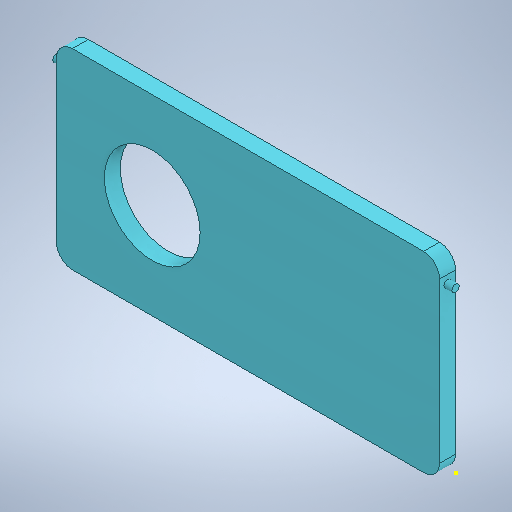
# Autodesk Inventor part: Puerta
Saved by Autodesk Inventor 2025.2 (Build 292293000, 293)
## iProperties
Created: 2024-11-26
Part Number: Puerta
Material: Plástico ABS
Document SubType Name: Modeling
Designer: usuario
Density: 1.06 g/cm^3
Appearance: Azul cadete
Author: usuario
Autodesk Inventor part; units mm, degrees
ref_plane "YZ Plane" through (0, 0, 0) normal (1, 0, 0) x (0, 1, 0)
ref_plane "XZ Plane" through (0, 0, 0) normal (0, 1, 0) x (-1, 0, 0)
sketch "Boceto1" plane through (0, 0, 0) normal (0, 0, 1) x (1, 0, 0)
  line L0 (5, 0) -> (115, 0)
  line L1 (120, 5) -> (120, 55)
  line L2 (115, 60) -> (5, 60)
  line L3 (0, 55) -> (0, 5)
  arc A0 (5, 60) -> (0, 55) centre (5, 55) ccw
  arc A1 (120, 55) -> (115, 60) centre (115, 55) ccw
  arc A2 (115, 0) -> (120, 5) centre (115, 5) ccw
  arc A3 (0, 5) -> (5, 0) centre (5, 5) ccw
  point P0 (0, 0)
  point P1 (120, 60)
  point P2 (120, 0)
  point P3 (0, 60)
  dimension "d0" = 120
  dimension "d1" = 60
  dimension "d2" = 5
  constraints: 8 end point, 8 point on circle, 8 point on line, 8 tangent, 4 centre point, 3 equal radius, 2 parallel, 1 horizontal, 1 perpendicular
  measures "d0" distance of point (0, 60) point (120, 60)
  measures "d1" distance of point (120, 60) point (120, 0)
  measures "d2" radius of A0
extrude "Extrusión1" add sketch "Boceto1" along normal blind 5
sketch "Boceto2" plane through (120, 5, 0) normal (1, 0, 0) x (0, 0, -1)
  point P0 (0, -5)
sketch "Boceto3" plane through (120, 5, 0) normal (1, 0, 0) x (0, 0, -1)
  circle A0 centre (-2.5, 47.5) radius 1.15
  line L0 (-5, 0) -> (-5, 50) projected
  line L1 (0, 50) -> (-5, 50) projected
  point P0 (0, -5)
  dimension "d5" = 2.3
  dimension "d6" = 2.5
  dimension "d7" = 2.5
  constraints: 1 centre point
  measures "d5" diameter of A0
  measures "d6" distance from line of L0 A0.centre
  measures "d7" distance from line of A0.centre L1
extrude "Extrusión2" add sketch "Boceto3" along normal blind 2.5
ref_plane "Plano de trabajo1" through (60, 5, 0) normal (1, 0, 0) x (0, 0, -1)
mirror "Simetría1" about plane through (60, 5, 0) normal (1, 0, 0) of "Extrusión2"
sketch "Boceto4" plane through (0, 0, 5) normal (0, 0, 1) x (1, 0, 0)
  circle A0 centre (30, 30) radius 15
  line L0 (0, 55) -> (0, 5) projected
  point P0 (0, 0)
  point P1 (0, 30)
  dimension "d10" = 30
  dimension "d11" = 30
  constraints: 1 centre point, 1 horizontal alignment, 1 midpoint
  measures "d10" diameter of A0
  measures "d11" distance from line of L0 A0.centre
extrude "Extrusión3" cut sketch "Boceto4" against normal through all
